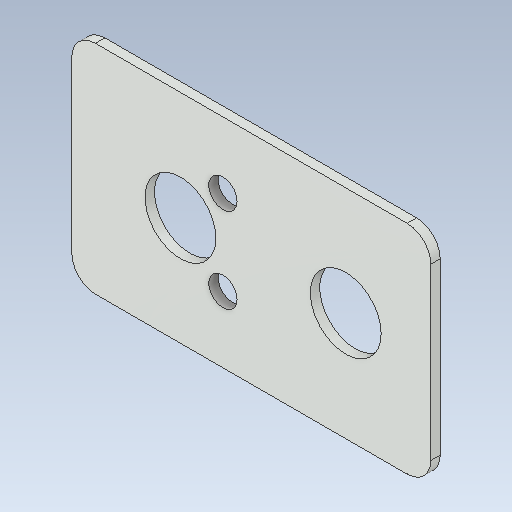
# Autodesk Inventor part: motor_acrylic_flange2
Saved by Autodesk Inventor 2020 (Build 240168000, 168)
## iProperties
Created: 2017-11-27
Part Number: motor_acrylic_flange2
Material: Generic
Document SubType Name: Modeling
Designer: stedrock
Density: 1 g/cm^3
Appearance: Default
Mass: 6.24222 g
Surface Area: 69.0155 cm^2
Volume: 6.24222 cm^3
Author: stedrock
Autodesk Inventor part; units mm, degrees
ref_plane "YZ Plane" through (0, 0, 0) normal (1, 0, 0) x (0, 1, 0)
ref_plane "XZ Plane" through (0, 0, 0) normal (0, 1, 0) x (-1, 0, 0)
ref_plane "XY Plane" through (0, 0, 0) normal (0, 0, 1) x (1, 0, 0)
sketch "Sketch1" plane through (0, 0, 0) normal (0, 0, 1) x (1, 0, 0)
  line L0 (-38, -23) -> (38, -23)
  line L1 (38, -23) -> (38, 23)
  line L2 (38, 23) -> (-38, 23)
  line L3 (-38, 23) -> (-38, -23)
  line L4 (-38, -23) -> (38, 23) construction
  line L5 (38, -23) -> (-38, 23) construction
  line L6 (0, 0) -> (42.6955, 0) construction
  circle A0 centre (20, 0) radius 7.5
  circle A1 centre (-15, 0) radius 7.5
  circle A2 centre (-6, 9) radius 3
  circle A3 centre (-6, -9) radius 3
  dimension "d0" = 76
  dimension "d1" = 46
  dimension "d2" = 15
  dimension "d5" = 20
  dimension "d7" = 15
  dimension "d8" = 35
  dimension "d9" = 6
  dimension "d10" = 9
  dimension "d11" = 9
  constraints: 14 end point, 4 centre point, 2 horizontal, 2 midpoint, 2 parallel, 1 perpendicular, 1 point on line, 1 symmetric about line, 1 other
  measures "d0" distance of L2.end L1.end
  measures "d1" distance of L1.end L0.end
  measures "d2" diameter of A0
  measures "d5" distance of L6.start A0.centre
  measures "d7" diameter of A1
  measures "d8" distance of A0.centre A1.centre
  measures "d9" diameter of A2
  measures "d10" vertical distance of L6.start A2.centre
  measures "d11" horizontal distance of A2.centre A1.centre
extrude "Extrusion1" add sketch "Sketch1" along normal blind 2
fillet "Fillet1" radius 5 4 edges at (-38, 23, 1) (38, 23, 1) (38, -23, 1) (-38, -23, 1)
body "Solid1"
